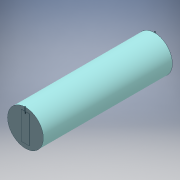
# Autodesk Inventor part: pila
Saved by Autodesk Inventor 2016 (Build 200138000, 138)
## iProperties
Created: 2017-12-28
Part Number: pila
Material: Genérico
Document SubType Name: Sheet Metal
Designer: David
Density: 1 g/cm^3
Sheet Metal Rule: Por defecto_mm
Appearance: Valor por defecto
Author: David
Autodesk Inventor part; units mm, degrees
ref_plane "YZ Plane" through (0, 0, 0) normal (1, 0, 0) x (0, 1, 0)
ref_plane "XZ Plane" through (0, 0, 0) normal (0, 1, 0) x (-1, 0, 0)
ref_plane "XY Plane" through (0, 0, 0) normal (0, 0, 1) x (1, 0, 0)
sketch "Boceto1" plane through (0, 0, 0) normal (0, 1, 0) x (-1, 0, 0)
  circle A0 centre (0, 0) radius 9
  constraints: 1 centre point, 1 coincident
extrude "Extrusión1" add sketch "Boceto1" along normal blind 32.5
sketch "Boceto3" plane through (0, 32.5, 0) normal (0, 1, 0) x (1, 0, 0)
  line L0 (-2, -7.1538) -> (2, -7.1538)
  line L1 (2, -7.1538) -> (2, 6.8462)
  line L2 (2, 6.8462) -> (-2, 6.8462)
  line L3 (-2, 6.8462) -> (-2, -7.1538)
  point P0 (0, 0)
  constraints: 8 end point, 2 parallel, 1 horizontal, 1 perpendicular
extrude "Extrusión2" add sketch "Boceto3" along normal blind 0.1
sketch "Boceto4" plane through (0, 32.6, 0) normal (0, 1, 0) x (1, 0, 0)
  line L0 (-2, -7.1538) -> (2, -7.1538) projected
  line L1 (-0.3, -7.1538) -> (-0.3, -6.2942)
  line L2 (-0.3, -6.2942) -> (0.3, -6.2942)
  line L3 (0.3, -6.2942) -> (0.3, -7.1538)
  line L4 (-0.1455, -7.1538) -> (-0.1455, -9.4777)
  line L5 (-0.1455, -9.4777) -> (0.146, -9.4777)
  line L6 (0.146, -9.4777) -> (0.146, -7.1538)
  line L7 (-0.3, -7.1538) -> (-0.1455, -7.1538)
  line L8 (0.146, -7.1538) -> (0.3, -7.1538)
  point P0 (0, 0)
  constraints: 16 end point, 4 perpendicular, 4 point on line, 2 horizontal, 2 vertical
extrude "Extrusión3" add sketch "Boceto4" along normal blind 0.2
fillet "Empalme1" radius 0.2 3 edges at (-0.3, 32.8, 6.724) (0.3, 32.8, 6.724) (0, 32.8, 6.2942)
fillet "Empalme2" radius 0.02 6 edges at (-0.1455, 32.6974, 9.4777) (0.146, 32.6974, 9.4777) (-0.1455, 32.6, 8.3158) (0.146, 32.6, 8.3158) (0.146, 32.7947, 8.3158) (-0.1455, 32.7949, 8.3158)
mirror "Simetría1" about plane through (0, 0, 0) normal (0, -1, 0) of "Extrusión1", "Extrusión3", "Extrusión2", "Empalme1"
equation "\"Radio_pliegue\" = Grosor"
equation "\"Anchura_desahogo_plegado\" = Grosor"
equation "\"Profundidad_desahogo_plegado\" = 0.5 * Grosor"
equation "\"Tamaño_destalonado\" = 4 * Grosor"
equation "\"Remanente_mínimo\" = 2 * Grosor"
equation "\"Radiodetransición\" = Radio_pliegue"
equation "\"Tamaño_de_radio_de_Jacobi\" = Radio_pliegue"
equation "\"TamañoSeparación\" = Grosor"
equation "\"Grosor\" = 0.5"
